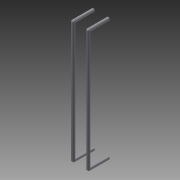
# Autodesk Inventor part: Y_Rail_Bridge-Rod-Rev1
Saved by Autodesk Inventor 2015 (Build 190159000, 159)
## iProperties
Created: 2016-12-21
Part Number: Y_Rail_Bridge-Rod-Rev1
Material: Generic
Document SubType Name: Modeling
Designer: Guy
Density: 1 g/cm^3
Appearance: Default
Author: Guy
Autodesk Inventor part; units mm, degrees
ref_plane "YZ Plane" through (0, 0, 0) normal (1, 0, 0) x (0, 1, 0)
ref_plane "XZ Plane" through (0, 0, 0) normal (0, 1, 0) x (-1, 0, 0)
ref_plane "XY Plane" through (0, 0, 0) normal (0, 0, 1) x (1, 0, 0)
sketch "Sketch1" plane through (0, 0, 0) normal (0, 0, 1) x (1, 0, 0)
  circle A0 centre (0, 0) radius 15
  circle A1 centre (150, 0) radius 15
  line L0 (0, 0) -> (150, 0)
  dimension "d0" = 30
  dimension "d3" = 30
  dimension "d4" = 150
  constraints: 2 centre point, 2 end point, 1 coincident, 1 horizontal
  measures "d0" diameter of A0
  measures "d3" diameter of A1
  measures "d4" distance of L0.end point (0, 0)
extrude "Extrusion1" add sketch "Sketch1" along normal blind 1200.8
sketch "Sketch2" plane through (0, 0, 0) normal (0, 1, 0) x (-1, 0, 0)
  line L0 (15, 1200.8) -> (-15, 1200.8) projected
  line L1 (-15, 0) -> (15, 0) projected
  line L2 (-135, 1200.8) -> (-165, 1200.8) projected
  line L3 (-165, 0) -> (-135, 0) projected
  circle A0 centre (0, 0) radius 15
  line L4 (-165, 0) -> (-135, 0) projected
  circle A1 centre (-150, 0) radius 15
  line L5 (15, 1200.8) -> (-15, 1200.8) projected
  circle A2 centre (0, 1200.8) radius 15
  line L6 (-135, 1200.8) -> (-165, 1200.8) projected
  circle A3 centre (-150, 1200.8) radius 15
  constraints: 4 horizontal alignment, 3 midpoint, 1 coincident, 8 other
extrude "Extrusion2" add sketch "Sketch2" along normal blind 200
sketch "Sketch3" plane through (0, 0, 1200.8) normal (0, 0, 1) x (1, 0, 0)
  line L0 (135, 0) -> (165, 0) projected
  line L1 (165, 0) -> (135, 0) projected
  arc A0 (135, 0) -> (165, 0) centre (150, 0) ccw projected
  line L2 (15, 0) -> (-15, 0) projected
  arc A1 (-15, 0) -> (15, 0) centre (0, 0) ccw projected
  circle A2 centre (150, 0) radius 15
  line L3 (165, 0) -> (135, 0)
  circle A3 centre (0, 0) radius 15
  line L4 (15, 0) -> (-15, 0)
  constraints: 4 end point, 2 centre point, 2 coincident, 2 concentric, 2 horizontal
revolve "Revolution1" add sketch "Sketch3" angle 90 about axis through (135, 0, 1200.8) along (-1, 0, 0) contours L0 A0 | A1 L2
body "Solid1"
